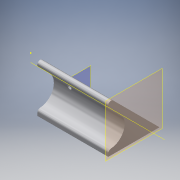
# Autodesk Inventor part: cutter
Saved by Autodesk Inventor 2019 (Build 230136000, 136)
## iProperties
Created: 2019-03-02
Part Number: cutter
Material: PET Plastic
Document SubType Name: Modeling
Designer: assman
Density: 1.541 g/cm^3
Appearance: Smooth - White
Author: assman
Autodesk Inventor part; units mm, degrees
ref_plane "YZ Plane" through (0, 0, 0) normal (1, 0, 0) x (0, 1, 0)
ref_plane "XZ Plane" through (0, 0, 0) normal (0, 1, 0) x (-1, 0, 0)
ref_plane "XY Plane" through (0, 0, 0) normal (0, 0, 1) x (1, 0, 0)
sketch "Sketch1" plane through (0, 0, 0) normal (1, 0, 0) x (0, 1, 0)
  line L0 (0, 0) -> (0, -19)
  line L1 (0, -19) -> (19, 0)
  line L2 (0, -19) -> (9.9437, -19) construction
  line L3 (0, -19) -> (19, 0)
  line L4 (19, 0) -> (0, 0)
  dimension "d0" = 19
  dimension "d1" = 45
  constraints: 10 end point, 2 horizontal, 1 coincident, 1 vertical
  measures "d0" distance of L0.end L0.start
  measures "d1" angle of L2 L1
extrude "Extrusion1" add sketch "Sketch1" along normal blind 61
sketch "Sketch2" plane through (61, 19, 0) normal (0, 0.7071068, -0.7071068) x (-1, 0, 0)
  line L0 (47, 0) -> (15, 0)
  line L1 (61, -26.8701) -> (0, -26.8701) projected
  line L2 (61, -26.8701) -> (0, -26.8701)
  line L3 (61, 0) -> (0, 0) projected
  line L4 (47, 0) -> (61, 0)
  line L5 (61, -26.8701) -> (61, 0) projected
  line L6 (61, 0) -> (61, -26.8701)
  line L7 (0, -26.8701) -> (0, 0) projected
  line L8 (0, 0) -> (0, -26.8701)
  line L9 (15, 0) -> (0, -26.8701)
  line L10 (47, 0) -> (61, -26.8701)
  point P0 (31, 0)
  point P1 (31, 0)
  dimension "d4" = 32
  constraints: 14 end point, 3 collinear, 1 horizontal, 1 midpoint, 1 perpendicular
  measures "d4" distance of L0.start L0.end
sketch "Sketch3" plane through (0, 0, 0) normal (-1, 0, 0) x (0, 0, 1)
  line L0 (-19, 0) -> (0, 19) projected
  line L1 (0, 19) -> (-12.7279, 6.2721)
  line L2 (-12.7279, 6.2721) -> (-9.8995, 3.4437)
  line L3 (-9.8995, 3.4437) -> (0, 13.3431)
  line L4 (0, 19) -> (0, 0) projected
  line L5 (-9.8995, 3.4437) -> (0, 3.4437)
  dimension "d5" = 18
  dimension "d6" = 4
  constraints: 8 end point, 3 perpendicular, 3 point on line
  measures "d5" distance of L0.end L1.end
  measures "d6" distance of L1.end L2.end
extrude "Extrusion2" cut sketch "Sketch3" against normal blind 62 contours L3 L4 L5
sketch "Sketch4" plane through (61, 0, -19) normal (0, 0.7071068, -0.7071068) x (-1, 0, 0)
  line L0 (61, 26.8701) -> (0, 26.8701) construction
  line L1 (30.5, 26.8701) -> (30.5, 0) construction
  line L2 (61, 0) -> (0, 0) construction
  line L3 (30.5, 17.2) -> (30.5, -1.6) construction
  line L4 (52.0668, -4.3668) -> (8.9332, 38.7668) construction
  line L5 (41.9599, 0) -> (41.9599, -16.3079)
  line L6 (41.9599, -16.3079) -> (-10.9063, -16.3079)
  line L7 (-10.9063, -16.3079) -> (-10.9063, 26.8701)
  line L8 (17.1357, 30.5643) -> (-10.9063, 30.5643)
  line L9 (-10.9063, 30.5643) -> (-10.9063, 26.8701)
  line L10 (17.1357, 30.5643) -> (41.9599, 30.5643)
  line L11 (41.9599, 0) -> (41.9599, 30.5643)
  line L12 (36.9964, -16.3079) -> (-5.0421, 25.7306)
  line L13 (-5.0421, 25.7306) -> (19.4362, 28.5467)
  line L14 (19.4362, 28.5467) -> (27.1412, 20.8416)
  line L15 (27.1412, 20.8416) -> (25.4088, 19.1092)
  arc A0 (25.4088, 19.1092) -> (27.6009, 16.9172) centre (26.5048, 18.0132) ccw
  line L16 (27.6009, 16.9172) -> (29.3333, 18.6496)
  line L17 (39.262, -16.3307) -> (41.8467, 6.1362)
  line L18 (29.3333, 18.6496) -> (31.9496, 16.0333)
  line L19 (31.9496, 16.0333) -> (30.2172, 14.3009)
  arc A1 (30.2172, 14.3009) -> (32.4092, 12.1088) centre (31.3132, 13.2048) ccw
  line L20 (32.4092, 12.1088) -> (34.1416, 13.8412)
  line L21 (34.1416, 13.8412) -> (41.8467, 6.1362)
  line L22 (29.1919, 18.5081) -> (29.3333, 18.6496)
  line L23 (29.3333, 18.6496) -> (29.4747, 18.5081)
  point P0 (61, 13.435)
  point P1 (47, 26.8701)
  point P2 (15, 26.8701)
  dimension "d13" = 18.8
  dimension "d14" = 1.6
  constraints: 44 end point, 5 point on line, 4 point on circle, 3 horizontal, 3 perpendicular, 2 centre point, 2 coincident, 2 collinear, 2 midpoint, 2 vertical
  measures "d13" distance of L3.start L3.end
  measures "d14" distance from line of L2 L3.end
extrude "Extrusion4" cut sketch "Sketch2" against normal blind 62 contours L3 L5 L10 | L9 L7 L3
sketch "Sketch5" plane through (61, 0, -19) normal (0, 0.7071068, -0.7071068) x (-1, 0, 0)
  point P0 (61, 13.435)
extrude "Extrusion5" add sketch "Sketch4" against normal up to surface (4 mm away)
sketch "Sketch6" plane through (19.0401, 0, -19) normal (-1, 0, 0) x (0, 0, 1)
  line L0 (-11.5314, -11.5314) -> (-5.8745, -11.5314)
  line L1 (5.6569, 0) -> (-5.8745, -11.5314)
  line L2 (-11.5314, -11.5314) -> (0, 0)
  line L3 (21.6122, 21.6122) -> (-11.5314, -11.5314) projected
  line L4 (19, 0) -> (0, 0) projected
  line L5 (5.6569, 0) -> (0, 0)
  line L6 (-11.5314, -11.5314) -> (-8.703, -14.3598) projected
  line L7 (-11.5314, -11.5314) -> (-8.703, -14.3598)
  line L8 (-8.703, -14.3598) -> (-5.8745, -11.5314)
  constraints: 12 end point, 2 collinear, 1 horizontal, 1 perpendicular, 1 point on line
extrude "Extrusion6" cut sketch "Sketch6" against normal blind 62 contours L0 L8 L6
ref_plane "Work Plane2" through (19.0401, 0, -19) normal (-1, 0, 0) x (0, 0, 1)
split "Split1" plane through (19.0401, 0, -19) removes the side toward (-1, 0, 0)
ref_plane "Work Plane3" through (19.0401, 18.7838, 5.4407) normal (0, -0.7071068, 0.7071068) x (1, 0, 0)
split "Split2" plane through (19.0401, 18.7838, 5.4407) removes the side toward (0, -0.7071068, 0.7071068)
sketch "Sketch7" plane through (19.0401, -11.5314, -30.5314) normal (-1, 0, 0) x (0, 0, 1)
  line L0 (5.6569, 0) -> (0, 0) projected
  line L1 (0, 0) -> (35, 0)
  line L2 (35, 0) -> (35, 4)
  line L3 (35, 4) -> (4, 4)
  line L4 (0, 0) -> (33.1436, 33.1436) projected
  line L5 (4, 4) -> (0, 0)
  point P0 (30.5314, 11.5314)
  dimension "d29" = 35
  dimension "d30" = 4
  constraints: 8 end point, 2 collinear, 2 perpendicular
  measures "d29" distance of L0.end L1.end
  measures "d30" distance of L1.end L2.end
extrude "Extrusion7" add sketch "Sketch7" against normal up to surface (52.8662 mm away)
sketch "Sketch8" plane through (71.9063, 21.6122, 2.6122) normal (0, 0.7071068, -0.7071068) x (-1, 0, 0)
  line L0 (30.3425, -2.0177) -> (38.0475, -9.7227)
  line L1 (62.973, -34.9311) -> (19.8395, 8.2024) construction
  line L2 (38.0475, -9.7227) -> (36.3151, -11.4551)
  arc A0 (36.3151, -11.4551) -> (38.5071, -13.6472) centre (37.4111, -12.5511) ccw
  line L3 (38.5071, -13.6472) -> (40.2395, -11.9147)
  line L4 (40.2395, -11.9147) -> (42.8558, -14.531)
  line L5 (42.8558, -14.531) -> (41.1234, -16.2635)
  arc A1 (41.1234, -16.2635) -> (43.3155, -18.4555) centre (42.2194, -17.3595) ccw
  line L6 (43.3155, -18.4555) -> (45.0479, -16.7231)
  line L7 (45.0479, -16.7231) -> (52.7529, -24.4281)
  line L8 (50.1709, -46.8722) -> (52.7529, -24.4281)
  line L9 (47.9026, -46.8722) -> (5.8642, -4.8337)
  line L10 (5.8642, -4.8337) -> (30.3425, -2.0177)
  line L11 (52.8662, -46.8722) -> (0, -46.8722)
  point P0 (71.9063, -17.1293)
  constraints: 24 end point, 4 point on circle, 2 centre point, 1 point on line
extrude "Extrusion8" cut sketch "Sketch8" against normal blind 0.2
fillet "Fillet1" radius 10 1 edges at (45.4732, -7.5314, -20.8745)
fillet "Fillet1" radius 2 3 edges at (45.4732, -7.5314, 4.4686) (45.4732, 18.7838, 5.4407) (45.4732, 21.6122, 2.6122)
sketch "Sketch9" plane through (71.9063, -11.5314, -30.5314) normal (0, 0.7071068, -0.7071068) x (-1, 0, 0)
  arc A0 (36.3151, 35.417) -> (38.5071, 33.225) centre (37.4111, 34.321) ccw projected
  point P0 (71.9063, 29.7429)
  constraints: 1 coincident
hole "Hole1" at (34.4952, 12.7372, -6.2628) direction (0, -0.7071068, 0.7071068) diameter 2.85 end through all
sketch "Sketch10" plane through (71.9063, -11.5314, -30.5314) normal (0, 0.7071068, -0.7071068) x (-1, 0, 0)
  arc A0 (41.1234, 30.6087) -> (43.3155, 28.4167) centre (42.2194, 29.5127) ccw projected
  point P0 (71.9063, 29.7429)
  constraints: 1 coincident
hole "Hole2" at (29.6868, 9.3372, -9.6628) direction (0, -0.7071068, 0.7071068) diameter 2.85 end through all
ref_plane "Work Plane4" through (66.9063, -11.5314, 4.4686) normal (1, 0, 0) x (0, 0, -1)
split "Split3" plane through (66.9063, -11.5314, 4.4686) removes the side toward (1, 0, 0)
sketch "Sketch11" plane through (19.0401, -11.5314, -30.5314) normal (-1, 0, 0) x (0, 0, 1)
  arc A0 (34.5578, 28.901) -> (31.7294, 31.7294) centre (33.1436, 30.3152) ccw projected
  line L0 (0, 0) -> (31.7294, 31.7294) projected
  line L1 (0, 0) -> (35, 0) projected
  line L2 (35, 0) -> (35, 2.0266) projected
  arc A1 (35, 2.0266) -> (33.1332, 4.0222) centre (33, 2.0266) ccw projected
  arc A2 (26.7279, 21.0711) -> (33.1332, 4.0222) centre (33.799, 14) ccw projected
  line L3 (26.7279, 21.0711) -> (34.5578, 28.901) projected
  point P0 (30.5314, 11.5314)
extrude "Extrusion9" add sketch "Sketch11" along normal blind 0.5
body "Solid1"
